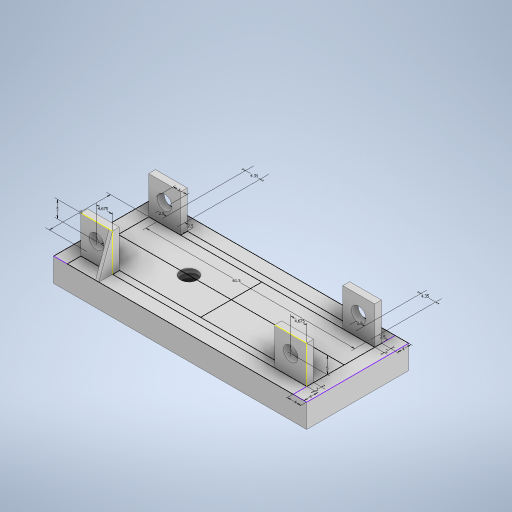
# Autodesk Inventor part: RadarMount
Saved by Autodesk Inventor 2023 (Build 270158000, 158)
## iProperties
Created: 2023-07-19
Part Number: RadarMount
Material: Generic
Document SubType Name: Modeling
Designer: beckb
Density: 1 g/cm^3
Appearance: Default
Author: beckb
## iProperties of the stored document RadarMount_3DPrint.ipt
Created: 2023-07-21
Part Number: RadarMount_3DPrint
Material: Generic
Document SubType Name: Modeling
Designer: beckb
Density: 1 g/cm^3
Appearance: Default
Author: beckb
Autodesk Inventor part; units mm, degrees
ref_plane "YZ Plane" through (0, 0, 0) normal (1, 0, 0) x (0, 1, 0)
ref_plane "XZ Plane" through (0, 0, 0) normal (0, 1, 0) x (-1, 0, 0)
ref_plane "XY Plane" through (0, 0, 0) normal (0, 0, 1) x (1, 0, 0)
sketch "Sketch1" plane through (0, 0, 0) normal (0, 1, 0) x (-1, 0, 0)
  line L0 (0, 0) -> (66.5, 0)
  line L1 (66.5, 0) -> (66.5, -22)
  line L2 (66.5, -22) -> (0, -22)
  line L3 (0, -22) -> (0, 0)
  line L4 (66.5, -2) -> (0, -2)
  line L5 (66.5, -20) -> (0, -20)
  line L6 (9.35, 0) -> (9.35, -2)
  line L7 (9.35, -20) -> (9.35, -22)
  line L8 (59.65, 0) -> (59.65, -2)
  line L9 (59.65, -20) -> (59.65, -22)
  line L10 (57.15, -22) -> (57.15, -20)
  line L11 (64, -22) -> (64, -20)
  line L12 (2.5, -22) -> (2.5, -20)
  line L13 (6.85, -22) -> (6.85, -20)
  line L14 (0, -11) -> (66.5, -11)
  line L15 (9.35, -2) -> (9.35, 0)
  line L16 (59.65, -2) -> (59.65, 0)
  line L17 (57.15, 0) -> (57.15, -2)
  line L18 (64, 0) -> (64, -2)
  line L19 (2.5, 0) -> (2.5, -2)
  line L20 (6.85, 0) -> (6.85, -2)
  line L21 (33.25, -2) -> (33.25, -20)
  line L22 (66.5, -22) -> (0, -22)
  line L23 (0, -22) -> (0, -26)
  line L24 (0, -26) -> (66.5, -26)
  line L25 (66.5, -26) -> (66.5, -22)
  line L26 (66.5, 0) -> (0, 0)
  line L27 (0, 0) -> (0, 4)
  line L28 (0, 4) -> (66.5, 4)
  line L29 (66.5, 4) -> (66.5, 0)
  line L30 (66.5, -26) -> (70.5, -26)
  line L31 (70.5, -26) -> (70.5, 4)
  line L32 (70.5, 4) -> (66.5, 4)
  line L33 (66.5, 4) -> (66.5, -26)
  line L34 (0, -26) -> (-4, -26)
  line L35 (-4, -26) -> (-4, 4)
  line L36 (-4, 4) -> (0, 4)
  line L37 (0, 4) -> (0, -26)
  point P0 (2.5, -21)
  point P1 (57.15, -21)
  point P2 (59.65, -21)
  point P3 (64, -21)
  point P4 (6.85, -21)
  point P5 (57.15, -2)
  point P6 (33.25, -11)
  point P7 (0, -22)
  point P8 (0, -22)
  dimension "d2" = 2
  dimension "d3" = 2
  dimension "d36" = 18
  dimension "d38" = 4.35
  dimension "d39" = 4.35
  dimension "d40" = 61.5
  dimension "d41" = 2.5
  dimension "d42" = 2.5
  dimension "d43" = 2.5
  dimension "d44" = 2.5
  dimension "d67" = 4
  dimension "d68" = 4
  dimension "d71" = 4
  dimension "d72" = 4
  constraints: 74 end point, 19 point on line, 10 parallel, 9 midpoint, 9 perpendicular, 8 symmetric about line, 5 horizontal, 5 vertical, 10 other
  measures "d3" distance between parallel lines of L0 L4
  measures "d38" distance of point (59.65, -21) point (64, -21)
  measures "d39" distance of point (2.5, -21) point (6.85, -21)
  measures "d40" distance between parallel lines of L11 L12
  measures "d41" distance between parallel lines of L12 L3
  measures "d42" distance between parallel lines of L1 L11
  measures "d43" distance between parallel lines of L10 L9
  measures "d44" distance between parallel lines of L13 L7
  measures "d67" distance of L22.end L23.end
  measures "d68" distance of L26.end L27.end
  measures "d71" distance of L24.end L30.end
  measures "d72" distance of L35.end L36.end
extrude "Extrusion2" add sketch "Sketch1" against normal blind 7 contours L0 L19 L4 L3 | L0 L20 L4 L19 | L4 L21 L14 L3 | L0 L6 L4 L20 | L14 L21 L5 L3 | L0 L17 L4 L6 | L5 L12 L2 L3 | L21 L4 L1 L14 | L14 L1 L5 L21 | L1 L4 L18 L0 | L0 L8 L4 L17 | L5 L13 L2 L12 | L5 L10 L2 L7 | L18 L4 L8 L0 | L5 L7 L2 L13 | L1 L2 L11 L5 | L5 L9 L2 L10 | L11 L2 L9 L5
extrude "Extrusion5" add sketch "Sketch1" along normal blind 11 contours L0 L19 L4 L3 | L0 L20 L4 L19 | L0 L6 L4 L20 | L5 L12 L2 L3 | L1 L4 L18 L0 | L0 L8 L4 L17 | L5 L13 L2 L12 | L18 L4 L8 L0 | L5 L7 L2 L13 | L1 L2 L11 L5 | L5 L9 L2 L10 | L11 L2 L9 L5
sketch "Sketch5" plane through (-66.5, -7, 0) normal (0, 0, 1) x (1, 0, 0)
  point P0 (66.5, 7)
sketch "Sketch6" plane through (-66.5, -7, 0) normal (0, 0, 1) x (1, 0, 0)
  point P0 (66.5, 7)
sketch "Sketch7" plane through (-66.5, -7, 0) normal (0, 0, 1) x (1, 0, 0)
  line L0 (66.5, 0) -> (66.5, 18) projected
  line L1 (57.15, 18) -> (66.5, 18) projected
  line L2 (0, 18) -> (9.35, 18) projected
  line L3 (9.35, 7) -> (9.35, 18) projected
  point P0 (66.5, 7)
  point P1 (61.825, 13)
  point P2 (4.675, 13)
  dimension "d55" = 4.675
  dimension "d56" = 5
  dimension "d57" = 5
  dimension "d58" = 4.675
  measures "d55" distance from line of L0 point (61.825, 13)
  measures "d56" distance from line of point (61.825, 13) L1
  measures "d57" distance from line of L2 point (4.675, 13)
  measures "d58" distance from line of L3 point (4.675, 13)
sketch "Sketch8" plane through (0, -7, -22) normal (0, 0, -1) x (-1, 0, 0)
  point P0 (0, 7)
  point P1 (4.675, 13)
  point P2 (61.825, 13)
hole "Hole3" at (-4.675, 6, -22) at (-61.825, 6, -22) direction (0, 0, 1) diameter 4.3 end through all
extrude "Extrusion6" add sketch "Sketch1" against normal blind 7 contours L27 L28 L29 L0 | L2 L25 L24 L23
extrude "Extrusion7" add sketch "Sketch1" against normal blind 7 contours L3 L23 L34 L35 L36 L27 | L32 L31 L30 L25 L1 L29
sketch "Sketch9" plane through (0, -7, 0) normal (0, -1, 0) x (1, 0, 0)
  line L0 (-70.5, 4) -> (4, 4) projected
  line L1 (4, -26) -> (-70.5, -26) projected
  line L2 (-70.5, -26) -> (-70.5, 4) projected
  line L3 (4, -26) -> (4, 4) projected
  line L4 (4, 4) -> (-70.5, 4) projected
  line L5 (-45.65, 4) -> (-45.65, -26)
  line L6 (-70.5, -11) -> (4, -11)
  line L7 (4, 4) -> (4, -26) projected
  point P0 (0, 0)
  point P1 (-33.25, -11)
  point P2 (-45.65, -11)
  dimension "d91" = 24.85
  constraints: 4 end point, 3 midpoint, 2 point on line, 1 perpendicular
  measures "d91" distance from line of point (-45.65, -11) L2
hole "Hole4" at (-45.65, -7, -11) direction (0, 1, 0) diameter 4.9784 end through all countersink diameter 7 countersink angle 135 thread size "1/4-20 UNC" class "1B" standard "ANSI Unified Screw Threads"
sketch "Sketch10" plane through (-57.15, 0, -2) normal (1, 0, 0) x (0, 0, -1)
  line L0 (-2, 0) -> (-2, 11) projected
  line L1 (-2, 11) -> (-6, 0)
  line L2 (-6, 0) -> (-2, 0)
  constraints: 4 end point, 1 horizontal
extrude "Extrusion8" add sketch "Sketch10" against normal blind 1
body "Solid1"
